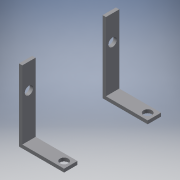
# Autodesk Inventor part: Fixação Caixa de Segurança
Saved by Autodesk Inventor 2019 (Build 230136000, 136)
## iProperties
Created: 2020-05-23
Part Number: Fixação Caixa de Segurança
Material: Genérico
Document SubType Name: Modeling
Designer: lukas
Density: 1 g/cm^3
Appearance: Padrão
Author: lukas
Autodesk Inventor part; units mm, degrees
ref_plane "YZ Plane" through (0, 0, 0) normal (1, 0, 0) x (0, 1, 0)
ref_plane "Plano de trabalho3" through (-51, -1, -36) normal (-1, 0, 0) x (0, 0, 1)
sketch "Esboço7" plane through (-51, -1, -36) normal (-1, 0, 0) x (0, 0, 1)
  circle A0 centre (61, 26) radius 2.5 projected
  line L0 (58.5, 41) -> (57, 41)
  line L1 (57, 41) -> (65, 41)
  line L2 (65, 41) -> (65, -2)
  line L3 (65, -2) -> (57, -2)
  line L4 (57, -2) -> (57, 41)
  line L5 (36, 36) -> (36, -3.986)
  circle A1 centre (11, 26) radius 2.5
  line L6 (15, 41) -> (7, 41)
  line L7 (7, 41) -> (7, -2)
  line L8 (7, -2) -> (15, -2)
  line L9 (15, -2) -> (15, 41)
  circle A2 centre (61, 26) radius 2.5
  point P0 (36, 1)
  dimension "d84" = 1.5
  dimension "d85" = 8
  dimension "d86" = 43
  dimension "d114" = 42
  dimension "d118" = 50
  constraints: 20 end point, 5 symmetric about line, 2 centre point, 2 horizontal, 2 parallel, 1 coincident, 1 concentric, 1 perpendicular, 1 vertical, 1 other
  measures "d84" distance of L0.start L0.end
  measures "d85" distance of L2.end L3.end
  measures "d86" distance of L1.end L2.end
  measures "d114" distance of L3.end L9.start
  measures "d118" distance of A0.centre A1.centre
extrude "Extrusão7" add sketch "Esboço7" along normal blind 2
ref_plane "Plano de trabalho6" through (0, -1, 0) normal (0, -1, 0) x (1, 0, 0)
sketch "Esboço8" plane through (0, -1, 0) normal (0, -1, 0) x (1, 0, 0)
  line L0 (-51, -29) -> (-36, -29)
  line L1 (-36, -29) -> (-36, -21)
  line L2 (-36, -21) -> (-51, -21)
  line L3 (-51, -21) -> (-51, -29)
  circle A0 centre (-40, 25) radius 2.5
  circle A1 centre (-40, -25) radius 2.5
  line L4 (-36, -25) -> (-40, -25)
  line L5 (-51, -21) -> (-51, -29) projected
  line L6 (-36, -21) -> (-51, -21)
  line L7 (-51, -21) -> (-51, -29)
  line L8 (-36, -24.068) -> (-36, -21)
  line L9 (-36, -21) -> (-51, -21)
  line L10 (-51, -21) -> (-51, -29)
  line L11 (-51, -29) -> (-36, -29)
  line L12 (-36, -29) -> (-36, -21)
  line L13 (-51, 21) -> (-53, 21) projected
  line L14 (-51, 21) -> (-26, 21)
  line L15 (-26, 21) -> (-26, 29)
  line L16 (-36.8, 29) -> (-61.8, 29)
  line L17 (-51, 29) -> (-51, 21)
  line L18 (-36, 21) -> (-36, 29)
  line L19 (-36, 25) -> (-40, 25)
  line L20 (-36, 29) -> (-51, 29)
  line L21 (-51, 29) -> (-51, 21)
  line L22 (-51, 21) -> (-36, 21)
  line L23 (-36, 21) -> (-36, 29)
  point P0 (0, 0)
  dimension "d90" = 15
  dimension "d116" = 4
  dimension "d119" = 8
  dimension "d120" = 4
  constraints: 44 end point, 9 parallel, 7 horizontal, 5 perpendicular, 3 point on line, 2 centre point, 2 midpoint
  measures "d90" distance of L2.end L1.end
  measures "d116" distance of L4.start L4.end
  measures "d119" distance of L15.end L14.end
  measures "d120" distance of L19.start L19.end
extrude "Extrusão8" add sketch "Esboço8" along normal blind 2
